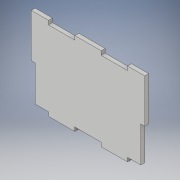
# Autodesk Inventor part: cham_back
Saved by Autodesk Inventor 2017.2 (Build 212233000, 233)
## iProperties
Created: 2017-06-02
Part Number: cham_back
Material: Generic
Document SubType Name: Modeling
Designer: SandeepSH
Density: 1 g/cm^3
Appearance: Default
Author: SandeepSH
Autodesk Inventor part; units mm, degrees
ref_plane "YZ Plane" through (0, 0, 0) normal (1, 0, 0) x (0, 1, 0)
ref_plane "XZ Plane" through (0, 0, 0) normal (0, 1, 0) x (-1, 0, 0)
ref_plane "XY Plane" through (0, 0, 0) normal (0, 0, 1) x (1, 0, 0)
sketch "Sketch1" plane through (0, 0, 0) normal (0, 0, 1) x (1, 0, 0)
  point P0 (0, 0)
sketch "Sketch2" plane through (0, 0, 0) normal (0, 0, 1) x (1, 0, 0)
  line L0 (-43, -31.5) -> (43, -31.5)
  line L1 (43, -31.5) -> (43, 31.5)
  line L2 (43, 31.5) -> (-43, 31.5)
  line L3 (-43, 31.5) -> (-43, -31.5)
  line L4 (-43, -31.5) -> (43, 31.5) construction
  line L5 (43, -31.5) -> (-43, 31.5) construction
  point P0 (0, 0)
  dimension "d0" = 86
  dimension "d1" = 63
  constraints: 12 end point, 2 midpoint, 2 parallel, 1 horizontal, 1 perpendicular
  measures "d0" distance of L2.end L1.end
  measures "d1" distance of L1.end L0.end
extrude "Extrusion1" add sketch "Sketch2" along normal blind 3
sketch "Sketch3" plane through (0, 0, 3) normal (0, 0, 1) x (1, 0, 0)
  line L0 (-43, -31.5) -> (43, -31.5) projected
  line L1 (-43, -31.5) -> (-40, -31.5)
  line L2 (-40, -31.5) -> (-40, -1.5)
  line L3 (-40, -1.5) -> (-43, -1.5)
  line L4 (-43, -1.5) -> (-43, -31.5)
  line L5 (43, -31.5) -> (40, -31.5)
  line L6 (40, -31.5) -> (40, -1.5)
  line L7 (40, -1.5) -> (43, -1.5)
  line L8 (43, -1.5) -> (43, -31.5)
  line L9 (-40, -31.5) -> (-30, -31.5)
  line L10 (-30, -31.5) -> (-30, -28.5)
  line L11 (-30, -28.5) -> (-40, -28.5)
  line L12 (-40, -28.5) -> (-40, -31.5)
  line L13 (40, -31.5) -> (30, -31.5)
  line L14 (30, -31.5) -> (30, -28.5)
  line L15 (30, -28.5) -> (40, -28.5)
  line L16 (40, -28.5) -> (40, -31.5)
  line L17 (-10, -31.5) -> (10, -31.5)
  line L18 (10, -31.5) -> (10, -28.5)
  line L19 (10, -28.5) -> (-10, -28.5)
  line L20 (-10, -28.5) -> (-10, -31.5)
  line L21 (43, 31.5) -> (-43, 31.5) projected
  line L22 (-30, 31.5) -> (-10, 31.5)
  line L23 (-10, 31.5) -> (-10, 28.5)
  line L24 (-10, 28.5) -> (-30, 28.5)
  line L25 (-30, 28.5) -> (-30, 31.5)
  line L26 (10, 31.5) -> (30, 31.5)
  line L27 (30, 31.5) -> (30, 28.5)
  line L28 (30, 28.5) -> (10, 28.5)
  line L29 (10, 28.5) -> (10, 31.5)
  point P0 (0, 0)
  dimension "d4" = 3
  dimension "d5" = 3
  dimension "d6" = 10
  dimension "d7" = 3
  dimension "d8" = 10
  dimension "d9" = 3
  dimension "d10" = 20
  dimension "d11" = 3
  dimension "d12" = 20
  dimension "d13" = 3
  dimension "d16" = 30
  constraints: 56 end point, 14 parallel, 7 horizontal, 7 perpendicular, 5 point on line
  measures "d4" distance of L3.end L2.end
  measures "d5" distance of L6.end L7.end
  measures "d6" distance of L11.end L10.end
  measures "d7" distance of L10.end L9.end
  measures "d8" distance of L14.end L15.end
  measures "d9" distance of L13.end L14.end
  measures "d10" distance of L19.end L18.end
  measures "d11" distance of L18.end L17.end
  measures "d12" distance between parallel lines of L14 L18
  measures "d13" distance of L22.end L23.end
  measures "d16" distance between parallel lines of L0 L3
extrude "Extrusion2" cut sketch "Sketch3" against normal through all
body "Solid1"
